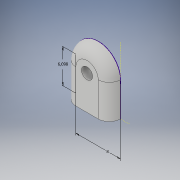
# Autodesk Inventor part: podpora_kciuk
Saved by Autodesk Inventor 2019 (Build 230136000, 136)
## iProperties
Created: 2020-01-12
Part Number: podpora_kciuk
Material: Ogólny
Document SubType Name: Modeling
Designer: Karolina
Density: 1 g/cm^3
Appearance: Domyślna
Author: Karolina
Autodesk Inventor part; units mm, degrees
ref_plane "YZ Plane" through (0, 0, 0) normal (1, 0, 0) x (0, 1, 0)
ref_plane "XZ Plane" through (0, 0, 0) normal (0, 1, 0) x (-1, 0, 0)
ref_plane "XY Plane" through (0, 0, 0) normal (0, 0, 1) x (1, 0, 0)
sketch "Szkic1" plane through (0, 0, 0) normal (0, 0, 1) x (1, 0, 0)
  line L0 (0, 12.1176) -> (0, -2.0196) construction
  line L1 (-9.6, 0) -> (1.6, 0) construction
  line L2 (0, 0) -> (-8, 0)
  line L3 (-8, 0) -> (-8, 6.098)
  line L4 (-8, 6.098) -> (0, 6.098)
  line L5 (0, 6.098) -> (0, 0)
  circle A0 centre (-4, 6.098) radius 4
  dimension "d0" = 8
  dimension "d1" = 6.098
  constraints: 8 end point, 2 parallel, 1 coincident, 1 horizontal, 1 horizontal alignment, 1 midpoint, 1 perpendicular, 2 other
  measures "d0" distance of L3.end L4.end
  measures "d1" distance of L2.end L3.end
extrude "Wyciągnięcie proste1" add sketch "Szkic1" along normal blind 2
hole "Otwór1" at (-4, 6.098, 0) direction (0, 0, 1) diameter 2 end through all
fillet "Zaokrąglenie1" radius 2 3 edges at (-4, 10.098, 2) (-8, 3.049, 2) (0, 3.049, 2)
